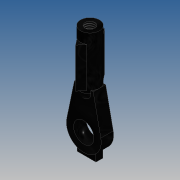
# Autodesk Inventor part: Rotule_M2
Saved by Autodesk Inventor 2021.3 (Build 253353000, 353)
## iProperties
Created: 2023-08-17
Part Number: Rotule_M2
Material: POM
Document SubType Name: Modeling
Designer: cedric.clivaz
Density: 1.425 g/cm^3
Appearance: Black
Author: cedric.clivaz
Autodesk Inventor part; units mm, degrees
ref_plane "YZ Plane" through (0, 0, 0) normal (1, 0, 0) x (0, 1, 0)
sketch "Sketch2" plane through (0, 0, 0) normal (0, 0, 1) x (1, 0, 0)
  circle A0 centre (0, 0) radius 1.9
  dimension "d0" = 3.8
  constraints: 1 centre point, 1 coincident
  measures "d0" diameter of A0
extrude "Extrusion1" add sketch "Sketch2" against normal blind 12.5
fillet "Fillet1" radius 1.9 1 edges at (-1.9, 0, -12.5)
sketch "Sketch3" plane through (0, 0, 0) normal (0, 1, 0) x (-1, 0, 0)
  line L0 (1.9, 0) -> (-1.9, 0) construction
  arc A0 (-3.4256, -17.2823) -> (3.4256, -17.2823) centre (0, -18) ccw
  line L1 (3.4256, -17.2823) -> (1.9, -10)
  line L2 (-3.4256, -17.2823) -> (-1.9, -10)
  line L3 (0, -27.6) -> (0, 4.6) construction
  line L4 (1.9, 0) -> (1.9, -10.6) construction
  line L5 (-1.9, 0) -> (-1.9, -10.6) construction
  line L6 (-1.9, -10) -> (1.9, -10)
  point P0 (0, 0)
  point P1 (-2.75, -11.75)
  point P2 (2.75, -11.75)
  dimension "d4" = 7
  dimension "d5" = 10
  dimension "d6" = 18
  dimension "d7" = 10
  constraints: 6 end point, 2 point on circle, 2 tangent, 1 centre point, 1 point on line, 4 other
  measures "d4" diameter of A0
  measures "d5" distance from line of L0 L1.end
  measures "d6" distance from line of L0 A0.centre
  measures "d7" distance from line of L0 L2.end
extrude "Extrusion2" add sketch "Sketch3" along normal mid plane 2.5
sketch "Sketch4" plane through (0, 0, 0) normal (0, 1, 0) x (-1, 0, 0)
  arc A0 (-3.4256, -17.2823) -> (3.4256, -17.2823) centre (0, -18) ccw construction
  arc A1 (-2.4, -18) -> (2.4, -18) centre (0, -18) ccw
  line L0 (2.4, -18) -> (-2.4, -18)
  point P0 (0, 0)
  dimension "d10" = 4.8
  constraints: 2 end point, 2 point on circle, 1 centre point, 1 coincident, 1 horizontal, 1 midpoint
  measures "d10" diameter of A1
revolve "Revolution1" cut sketch "Sketch4" angle 360 about axis through (-2.4, 0, -18) along (1, 0, 0)
sketch "Sketch5" plane through (0, 0, 0) normal (0, 0, 1) x (1, 0, 0)
  circle A0 centre (0, 0) radius 1
  dimension "d12" = 2
  constraints: 1 centre point, 1 coincident
  measures "d12" diameter of A0
extrude "Extrusion3" cut sketch "Sketch5" against normal blind 12
thread "Thread1" size "M2x0.4" designation "M2" class "6H" standard "ISO Metric profile" length 110
ref_plane "Work Plane1" through (0, 0, -21.5) normal (0, 0, 1) x (1, 0, 0)
sketch "Sketch6" plane through (0, 0, -21.5) normal (0, 0, 1) x (1, 0, 0)
  line L0 (-4.9, 0) -> (4.9, 0) construction
  line L1 (0, -2.66) -> (0, 2.66) construction
  line L2 (1.9, 0.7) -> (-1.9, 0.7)
  line L3 (-1.9, 0.7) -> (-1.9, -0.7)
  line L4 (-1.9, -0.7) -> (1.9, -0.7)
  line L5 (1.9, -0.7) -> (1.9, 0.7)
  point P0 (0, 0)
  dimension "d17" = 3.8
  dimension "d18" = 1.4
  constraints: 8 end point, 2 parallel, 1 horizontal, 1 perpendicular, 2 other
  measures "d17" distance of L4.end L3.end
  measures "d18" distance of L3.end L2.end
extrude "Extrusion4" add sketch "Sketch6" against normal blind 1
sketch "Sketch7" plane through (0, 0, -21.5) normal (0, 0, 1) x (1, 0, 0)
  line L0 (-1.9, -0.7) -> (-1.9, 0.7) construction
  line L1 (-1.9, 0.7) -> (1.9, 0.7) construction
  line L2 (1.9, 0.7) -> (1.9, -0.7) construction
  line L3 (1.9, -0.7) -> (-1.9, -0.7) construction
  line L4 (-1.9, 0.7) -> (1.9, 0.7)
  line L5 (1.9, 0.7) -> (1.9, -0.7)
  line L6 (1.9, -0.7) -> (-1.9, -0.7)
  line L7 (-1.9, -0.7) -> (-1.9, 0.7)
  point P0 (0, 0)
  constraints: 8 end point, 2 parallel, 1 horizontal, 1 perpendicular
extrude "Extrusion5" add sketch "Sketch7" along normal up to surface
ref_plane "Work Plane2" through (0, 0, -2) normal (0, 0, 1) x (1, 0, 0)
sketch "Sketch8" plane through (0, 0, -2) normal (0, 0, 1) x (1, 0, 0)
  arc A0 (1.4309, 1.25) -> (-1.4309, 1.25) centre (0, 0) ccw construction
  circle A1 centre (0, 0) radius 1.9
  line L0 (0, -2.98) -> (0, 4.58) construction
  line L1 (-2.66, 0) -> (2.66, 0) construction
  line L2 (-1, 1.6155) -> (0, 2.9)
  line L3 (1, 1.6155) -> (0, 2.9)
  dimension "d24" = 2.9
  dimension "d25" = 2
  constraints: 4 end point, 2 point on circle, 1 centre point, 1 coincident, 1 concentric, 1 point on line, 1 symmetric about line
  measures "d24" distance from line of L2.end L1
  measures "d25" distance of L3.start L2.start
extrude "Extrusion6" add sketch "Sketch8" against normal blind 8 contours A1 L2 L3
mirror "Mirror1" about plane through (0, 0, 0) normal (0, 1, 0) of "Extrusion6"
equation "\"d5\" = d7"
body "Solid1"
